skadis_nut_right (Autodesk Fusion 360 design; units mm, degrees)
part number: 2026-09-06-14-40-23-923
Autodesk Fusion 360 part; units mm, degrees
sketch "Plate" plane through (0, 0, 0) normal (0, 1, 0) x (1, 0, 0)
  line L0 (0, 0) -> (11, 0)
  line L1 (11, 0) -> (11, -48)
  line L2 (11, -48) -> (0, -48)
  line L3 (0, -48) -> (0, 0)
  dimension "d175" = 11
  dimension "d176" = 48
  constraint coincident L0.start L3.end
  constraint horizontal L0
  constraint horizontal L2
  constraint vertical L1
  constraint vertical L3
  measures "d175" horizontal distance of L0.start L1.end
  measures "d176" vertical distance of L0.start L1.end
extrude "Plate (1)" add sketch "Plate" along normal mid plane 33 from surface at -4.5
sketch "Hook profile" plane through (0, 0, 0) normal (0, 1, 0) x (1, 0, 0)
  line L0 (0, -46) -> (-8.3, -46)
  line L1 (-8.3, -46) -> (-8.3, -29)
  line L2 (-8.3, -29) -> (-5.3, -29)
  line L3 (-5.3, -29) -> (-3.8, -30.5)
  line L4 (-3.8, -30.5) -> (-3.8, -41)
  line L5 (-3.8, -41) -> (0, -41)
  line L6 (0, -41) -> (0, -46)
  dimension "d180" = 46
  dimension "d181" = 8.3
  dimension "d182" = 3.8
  dimension "d183" = 5
  dimension "d184" = 10.5
  dimension "d185" = 1.5
  dimension "d186" = 1.5
  constraint horizontal L0
  constraint horizontal L2
  constraint horizontal L5
  constraint vertical L1
  constraint vertical L4
  constraint vertical L6
  constraint coincident origin L6
  measures "d180" vertical distance of origin L0.start
  measures "d181" horizontal distance of L0.start L0.end
  measures "d182" horizontal distance of L4.end L5.end
  measures "d183" vertical distance of L0.start L5.end
  measures "d184" vertical distance of L3.end L4.end
  measures "d185" horizontal distance of L2.end L3.end
  measures "d186" vertical distance of L2.end L3.end
extrude "Hook profile (1)" add sketch "Hook profile" along normal mid plane 2.4
pattern_linear "Hook rows" count 2 spacing 25.4 along (0, 0, -1) count 3 spacing 0 along (0, 0, 1) of "Hook profile (1)"
sketch "Screw hole" plane through (0, 0, 0) normal (0, 1, 0) x (1, 0, 0)
  line L0 (-1, -21.6) -> (12, -21.6)
  line L1 (12, -21.6) -> (12, -26.4)
  line L2 (12, -26.4) -> (-1, -26.4)
  line L3 (-1, -26.4) -> (-1, -21.6)
  dimension "d193" = 12
  dimension "d194" = 21.6
  dimension "d195" = 13
  dimension "d196" = 4.8
  constraint horizontal L0
  constraint horizontal L2
  constraint vertical L1
  constraint vertical L3
  measures "d193" horizontal distance of origin L0.end
  measures "d194" vertical distance of origin L0.end
  measures "d195" horizontal distance of L0.start L0.end
  measures "d196" vertical distance of L0.end L1.end
extrude "Screw hole (1)" cut sketch "Screw hole" along normal mid plane 16.8 from surface at -7.52
sketch "Nut cavity" plane through (0, 0, 0) normal (0, 1, 0) x (1, 0, 0)
  line L0 (4.5, -20.3) -> (7, -20.3)
  line L1 (7, -20.3) -> (7, -27.7)
  line L2 (7, -27.7) -> (4.5, -27.7)
  line L3 (4.5, -27.7) -> (4.5, -20.3)
  dimension "d200" = 7
  dimension "d201" = 20.3
  dimension "d202" = 2.5
  dimension "d203" = 7.4
  constraint horizontal L0
  constraint horizontal L2
  constraint vertical L1
  constraint vertical L3
  measures "d200" horizontal distance of origin L0.end
  measures "d201" vertical distance of origin L0.end
  measures "d202" horizontal distance of L0.start L0.end
  measures "d203" vertical distance of L0.end L1.end
extrude "Nut cavity (1)" cut sketch "Nut cavity" along normal mid plane 30.22 from surface at -2.11
equation "bracketWidth = 24.0 mm" comment "bracket width across the upright"
equation "plateHeight = 48.0 mm" comment "plate height"
equation "plateInboardExtension = 9.0 mm" comment "extra plate toward the desk centre, where the channel reaches"
equation "boardThickness = 6.0 mm" comment "measured SKADIS panel thickness"
equation "screwLength = 15.0 mm" comment "measured decorative M4 screw"
equation "screwDiameter = 4.0 mm" comment "M4 shank"
equation "screwClearance = 0.8 mm" comment "slack around the shank"
equation "screwTipClearance = 2.0 mm" comment "tip stops this short of the plate's back face"
equation "screwSlotWidth = screwDiameter + screwClearance" comment "screw relief slot height"
equation "nutAcrossFlats = 7.0 mm" comment "M4 square nut across flats"
equation "nutThickness = 2.2 mm" comment "M4 square nut thickness"
equation "nutChannelClearance = 0.4 mm" comment "slack around the nut in its channel"
equation "nutChannelHeight = nutAcrossFlats + nutChannelClearance" comment "channel height; under the nut's diagonal so it cannot turn"
equation "plateThickness = screwLength - boardThickness + screwTipClearance" comment "derived: deep enough to swallow the screw"
equation "mountTravel = 12.0 mm" comment "left-right adjustment"
equation "nutChannelLength = mountTravel + nutAcrossFlats + nutChannelClearance" comment "channel length along the plate"
equation "screwSlotLength = mountTravel + screwSlotWidth" comment "relief slot length along the plate"
equation "topMountZ = 24.0 mm" comment "top channel centre"
equation "mountOffsetY = -7.52 mm" comment "channel centre on the board's grid"
equation "slotOvershoot = 1.0 mm" comment "cuts reach past the faces they cut"
equation "slotWidth = 3.2 mm" comment "measured upright slot width"
equation "slotPitchVertical = 25.4 mm" comment "1 inch, measured"
equation "faceMetalThickness = 2.0 mm" comment "upright face metal"
equation "hookTabWidth = slotWidth - 0.8 mm" comment "blade width through the slot"
equation "hookThroat = faceMetalThickness + 1.8 mm" comment "gap behind the plate"
equation "hookNeckHeight = 5.0 mm" comment "bears on the slot bottom edge"
equation "hookLipThickness = 4.5 mm" comment "lip behind the upright face"
equation "hookLipDrop = 12.0 mm" comment "engagement below the neck"
equation "hookLipChamfer = 1.5 mm" comment "lead-in past slot burrs"
equation "topHookNeckTop = plateHeight - 2 mm" comment "top hook row"
equation "hookRows = 2" comment "hook rows (pattern count)"
equation "nutCavityClearance = 0.3 mm" comment "slack across the nut's thickness"
equation "nutWallThickness = 4.0 mm" comment "wall in front of the nut; the screw pulls the nut against it"
equation "nutCavityDepth = nutThickness + nutCavityClearance" comment "cavity depth"
equation "d175 = plateThickness"
equation "d176 = plateHeight"
equation "d177 = -plateInboardExtension / 2"
equation "d178 = bracketWidth + plateInboardExtension"
equation "d180 = topHookNeckTop"
equation "d181 = hookThroat + hookLipThickness"
equation "d182 = hookThroat"
equation "d183 = hookNeckHeight"
equation "d184 = hookLipDrop - hookLipChamfer"
equation "d185 = hookLipChamfer"
equation "d186 = hookLipChamfer"
equation "d187 = hookTabWidth"
equation "d189 = hookRows"
equation "d191 = -slotPitchVertical"
equation "d193 = plateThickness + slotOvershoot"
equation "d194 = topMountZ - screwSlotWidth / 2"
equation "d195 = plateThickness + 2 * slotOvershoot"
equation "d196 = screwSlotWidth"
equation "d197 = mountOffsetY"
equation "d198 = screwSlotLength"
equation "d200 = plateThickness - nutWallThickness"
equation "d201 = topMountZ - nutChannelHeight / 2"
equation "d202 = nutCavityDepth"
equation "d203 = nutChannelHeight"
equation "d204 = ( mountOffsetY - nutChannelLength / 2 + bracketWidth / 2 + slotOvershoot ) / 2"
equation "d205 = -mountOffsetY + nutChannelLength / 2 + bracketWidth / 2 + slotOvershoot"
named bodies: "skadis_nut_right"
